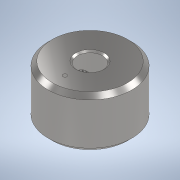
# Autodesk Inventor part: Pendulum Arm Cap
Saved by Autodesk Inventor 2021.1 (Build 251245010, 245A)
## iProperties
Created: 2025-09-16
Part Number: Pendulum Arm Cap
Material: Stainless Steel
Document SubType Name: Modeling
Designer: SD
Density: 8 g/cm^3
Appearance: Semi-Polished
Mass: 3.2247 g
Surface Area: 3.85637 cm^2
Volume: 0.403087 cm^3
Project: Automatic Tea Steeping mechanism
Length: 6.000 mm
BOM-Mass: 0.00322
BOM-Area: 0.000
Diameter: 10.000 mm
Author: SD
Title: Pendulum Arm Cap
Autodesk Inventor part; units mm, degrees
ref_plane "YZ Plane" through (0, 0, 0) normal (1, 0, 0) x (0, 1, 0)
ref_plane "XZ Plane" through (0, 0, 0) normal (0, 1, 0) x (-1, 0, 0)
ref_plane "XY Plane" through (0, 0, 0) normal (0, 0, 1) x (1, 0, 0)
sketch "Sketch1" plane through (0, 0, 0) normal (0, 1, 0) x (-1, 0, 0)
  circle A0 centre (0, 0) radius 5
  dimension "Diameter" = 10
  constraints: 1 centre point, 1 coincident
  measures "Diameter" diameter of A0
extrude "Extrusion1" add sketch "Sketch1" along normal mid plane 6
sketch "Sketch2" plane through (0, 3, 0) normal (0, 1, 0) x (1, 0, 0)
  circle A0 centre (0, 0) radius 1.5
  dimension "d3" = 3
  constraints: 1 centre point, 1 coincident
  measures "d3" diameter of A0
extrude "Extrusion2" cut sketch "Sketch2" against normal through all
sketch "Sketch3" plane through (0, 0, 0) normal (1, 0, 0) x (0, 1, 0)
  circle A0 centre (0, 0) radius 1.25
  dimension "d6" = 2.5
  constraints: 1 centre point, 1 coincident
  measures "d6" diameter of A0
extrude "Extrusion3" cut sketch "Sketch3" against normal blind 6
chamfer "Chamfer1" distance 0.5 angle 45 2 edges at (5, 3, 0) (5, -3, 0)
chamfer "Chamfer2" distance 0.2 angle 45 2 edges at (-1.5, 3, 0) (-1.5, -3, 0)
thread "Thread1" size "M3x0.5" class "6H" standard "ANSI Metric M Profile" length 5
sketch "Sketch4" plane through (0, 3, 0) normal (0, 1, 0) x (1, 0, 0)
  point P0 (0, 0)
  point P1 (0, -3)
  dimension "d17" = 3
  constraints: 1 vertical alignment
  measures "d17" distance of point (0, -3) point (0, 0)
hole "Hole1" at (0, 3, 3) direction (0, -1, 0) diameter 0.5 end through all
body "Solid1"
